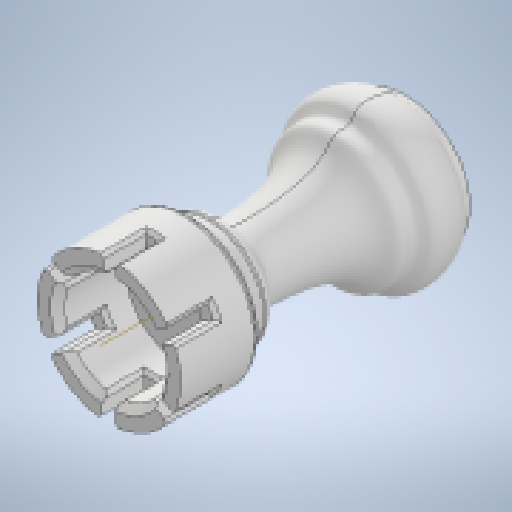
# Autodesk Inventor part: rook-white
Saved by Autodesk Inventor 2024.1 (Build 281209000, 209)
## iProperties
Created: 2025-08-03
Part Number: rook-white
Material: Generic
Document SubType Name: Modeling
Designer: iwheard
Density: 1 g/cm^3
Appearance: Default
Author: iwheard
Autodesk Inventor part; units mm, degrees
ref_plane "YZ Plane" through (0, 0, 0) normal (1, 0, 0) x (0, 1, 0)
ref_plane "XZ Plane" through (0, 0, 0) normal (0, 1, 0) x (-1, 0, 0)
ref_plane "XY Plane" through (0, 0, 0) normal (0, 0, 1) x (1, 0, 0)
sketch "Sketch1" plane through (0, 0, 0) normal (0, 0, 1) x (1, 0, 0)
  circle A0 centre (0, 25.5) radius 3
  circle A1 centre (0, 25.5) radius 5
  point P0 (0, 0)
  dimension "d0" = 10
  constraints: 2 centre point
  measures "d0" diameter of A1
extrude "Extrusion1" add sketch "Sketch1" along normal blind 3
sketch "Sketch3" plane through (0, 25.5, 3) normal (0, 0, 1) x (1, 0, 0)
  circle A0 centre (0, 0) radius 5 projected
  circle A1 centre (0, 0) radius 3 projected
  circle A2 centre (0, 0) radius 7.15
  point P0 (0, -25.5)
  dimension "d6" = 14.3
  constraints: 1 centre point
  measures "d6" diameter of A2
extrude "Extrusion2" add sketch "Sketch3" against normal blind 3 contours A2
sketch "Sketch2" plane through (0, 0, 0) normal (1, 0, 0) x (0, 1, 0)
  line L0 (30.5, 3) -> (20.5, 3) projected
  line L1 (30.5, 0) -> (20.5, 0) projected
  line L2 (30.5, 0) -> (30.5, 3) projected
  line L3 (28.5, 3) -> (28.5, 0) projected
  line L4 (32.65, 3) -> (18.35, 3) projected
  line L5 (32.65, 3) -> (32.65, 0) projected
  line L6 (32.65, 0.8) -> (33.5351, 1.2027) construction
  line L7 (33.5351, 1.2027) -> (34.0973, 2.2554) construction
  line L8 (34.0973, 2.2554) -> (34.5096, 4.0365) construction
  line L9 (34.5096, 4.0365) -> (34.2463, 5.2149) construction
  line L10 (34.2463, 5.2149) -> (33.8162, 5.9148) construction
  line L11 (33.8162, 5.9148) -> (33.1018, 6.0655) construction
  line L12 (33.1018, 6.0655) -> (32.6685, 6.8872) construction
  line L13 (32.6685, 6.8872) -> (33.459, 8.43) construction
  line L14 (33.459, 8.43) -> (29.9033, 9.0192) construction
  line L15 (29.9033, 9.0192) -> (29.3908, 18.4815) construction
  line L16 (31.7, 22) -> (31.7, 22) construction
  spline S0 degree 4 poles (32.65, 0.8) (33.5351, 1.2027) (34.0973, 2.2554) (34.5096, 4.0365) (34.2463, 5.2149) (33.8162, 5.9148) (33.1018, 6.0655) (32.6685, 6.8872) (33.459, 8.43) (29.9033, 9.0192) (29.3908, 18.4815) (29.5859, 19.8436) (31.1715, 20.6812) (31.6218, 21.262) (31.6999, 21.9993) (31.7, 22) knots 1 1 1 1 1 2 3 4 5 6 7 8 9 10 10.505813 10.92418 11 11 11 11 11
  line L17 (31.6218, 21.262) -> (31.7, 22) construction
  line L18 (29.3908, 18.4815) -> (29.5859, 19.8436) construction
  line L19 (29.5859, 19.8436) -> (31.1715, 20.6812) construction
  line L20 (31.1715, 20.6812) -> (31.6218, 21.262) construction
  line L21 (25.5, -8.48) -> (25.5, 50.88) projected
  line L22 (31.7, 22) -> (25.5, 22)
  line L23 (31.58, 22) -> (32.4653, 23.8)
  line L24 (32.6653, 23.8) -> (33.5, 24.7)
  line L25 (33.5, 24.7) -> (25.5, 24.7)
  line L26 (25.5, 24.7) -> (25.5, 33.1)
  line L27 (25.5, 33.1) -> (33.5, 33.1)
  line L28 (33.5, 33.1) -> (33.5, 24.7)
  line L29 (32.6653, 23.8) -> (32.4653, 23.8)
  point P0 (0, 0)
  point P1 (25.5, 3)
  point P2 (25.5, 0)
  point P3 (25.5, 3)
  dimension "d135" = 0.8
  dimension "d146" = 22
  dimension "d147" = 6.2
  dimension "d151" = 8
  dimension "d152" = 33.1
  dimension "d153" = 8.4
  dimension "d154" = 0.2
  dimension "d155" = 1.8
  constraints: 16 end point, 3 horizontal alignment, 3 midpoint, 1 coincident, 1 horizontal, 1 point on line, 1 vertical alignment, 5 other
  measures "d135" distance from line of L6.start L1
  measures "d146" distance from line of L16.end L1
  measures "d147" distance from line of L21 L16.end
  measures "d151" distance between parallel lines of L26 L28
  measures "d152" distance between parallel lines of L1 L27
  measures "d153" distance between parallel lines of L25 L27
  measures "d154" distance of L23.end L24.start
  measures "d155" distance from line of L16.end L29
revolve "Revolution1" add sketch "Sketch2" angle 360 about axis through (0, 25.5, 0) along (0, 0, 1) contours L0 L21 L22 S0 L5 L4 | L21 L25 L24 L29 L23 L22 | L21 L27 L28 L25
sketch "Sketch18" plane through (0, 25.5, 33.1) normal (0, 0, 1) x (1, 0, 0)
  circle A0 centre (0, 0) radius 3 projected
  circle A1 centre (0, 0) radius 5.75
  point P0 (0, -25.5)
  dimension "d156" = 11.5
  constraints: 1 centre point
  measures "d156" diameter of A1
extrude "Extrusion12" cut sketch "Sketch18" against normal blind 7.65 contours A0 | A1
sketch "Sketch19" plane through (0, 25.5, 33.1) normal (0, 0, 1) x (1, 0, 0)
  line L0 (-0.5896, 10.7302) -> (0.8105, 10.7302)
  line L1 (0.8105, 10.7302) -> (0.5733, -12.3151)
  line L2 (0.5733, -12.3151) -> (-0.8268, -12.3151)
  line L3 (-0.8268, -12.3151) -> (-0.5896, 10.7302)
  point P0 (0, -25.5)
  point P1 (0, 0)
  dimension "d159" = 1.4
  dimension "d160" = 0.7
  constraints: 8 end point
  measures "d159" distance between parallel lines of L1 L3
  measures "d160" distance from line of L3 point (0, 0)
extrude "Extrusion13" cut sketch "Sketch19" against normal blind 4.73
pattern_circular "Circular Pattern6" count 3 over 360 about axis through (0, 25.5, 0) along (0, 0, 1) of "Extrusion13"
fillet "Fillet9" radius 0.5 1 edges at (0, 17.5, 24.7)
fillet "Fillet10" radius 0.5 1 edges at (0, 18.3347, 23.8)
fillet "Fillet11" radius 0.2 1 edges at (0, 19.3, 22)
chamfer "Chamfer7" distance 0.4 angle 45 18 edges at (-0.6412, 31.2141, 30.735) (0.0592, 31.2497, 28.37) (0.7587, 31.1997, 30.735) (-4.5568, 29.0069, 30.735) (-5.2692, 27.8017, 30.735) (-4.9498, 28.4261, 28.37) (5.009, 28.3236, 28.37) (4.628, 28.9124, 30.735) (5.3155, 27.6928, 30.735) (-5.009, 22.6764, 28.37) (-5.3155, 23.3072, 30.735) (-4.628, 22.0876, 30.735) (-0.0592, 19.7503, 28.37) (-0.7587, 19.8003, 30.735) (0.6412, 19.7859, 30.735) (5.2692, 23.1983, 30.735) (4.9498, 22.5739, 28.37) (4.5568, 21.9931, 30.735)
chamfer "Chamfer8" distance 0.4 angle 45 19 edges at (-0.0823, 17.5004, 28.37) (-0.782, 17.5383, 30.735) (0.618, 17.5239, 30.735) (-6.5985, 20.9768, 30.735) (-6.969, 21.5715, 28.37) (-7.286, 22.1964, 30.735) (6.8867, 21.4289, 28.37) (6.504, 20.842, 30.735) (7.2165, 22.0471, 30.735) (7.286, 28.8036, 30.735) (6.5985, 30.0232, 30.735) (6.969, 29.4285, 28.37) (-0.618, 33.4761, 30.735) (0.3915, 33.4904, 28.37) (-0.3092, 33.494, 28.37) (0.782, 33.4617, 30.735) (-6.504, 30.158, 30.735) (-7.2165, 28.9529, 30.735) (-6.8867, 29.5711, 28.37)
chamfer "Chamfer9" distance 0.8 angle 45 7 edges at (-5.7497, 25.5592, 33.1) (-2.9261, 20.5502, 33.1) (-2.8236, 30.509, 33.1) (2.9261, 30.4498, 33.1) (5.6758, 26.4209, 33.1) (5.666, 24.5208, 33.1) (2.8236, 20.491, 33.1)
body "Solid1"
